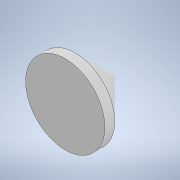
# Autodesk Inventor part: extruderHead
Saved by Autodesk Inventor 2020 (Build 240168000, 168)
## iProperties
Created: 2020-07-15
Part Number: extruderHead
Material: Generic
Document SubType Name: Modeling
Designer: zhang
Density: 1 g/cm^3
Appearance: Default
Author: zhang
Autodesk Inventor part; units mm, degrees
ref_plane "YZ Plane" through (0, 0, 0) normal (1, 0, 0) x (0, 1, 0)
ref_plane "XZ Plane" through (0, 0, 0) normal (0, 1, 0) x (-1, 0, 0)
ref_plane "XY Plane" through (0, 0, 0) normal (0, 0, 1) x (1, 0, 0)
sketch "Sketch4" plane through (0, 0, 0) normal (0, 1, 0) x (-1, 0, 0)
  line L0 (0, 100) -> (-80, 100)
  line L1 (-80, 100) -> (-80, 80)
  line L2 (-80, 80) -> (0, 0)
  line L3 (0, 0) -> (0, 100)
  dimension "d7" = 80
  dimension "d8" = 100
  dimension "d12" = 80
  constraints: 8 end point, 1 horizontal, 1 parallel, 1 perpendicular
  measures "d7" distance of L0.start L0.end
  measures "d8" distance of L2.end L0.start
  measures "d12" horizontal distance of L1.end L2.end
revolve "Revolution2" add sketch "Sketch4" angle 360 about axis through (0, 0, 0) along (0, 0, 1)
body "Solid3"
